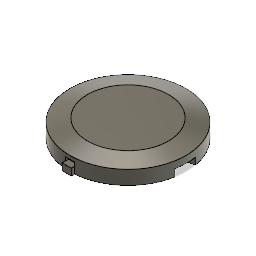
CaseBack (Autodesk Fusion 360 design; units mm, degrees)
Autodesk Fusion 360 part; units mm, degrees
sketch "Sketch1" plane through (0, 0, 0) normal (0, 1, 0) x (1, 0, 0)
  circle A0 centre (0, 0) radius 16.4
  dimension "d1" = 32.8
  measures "d1" diameter of A0
extrude "Extrude1" add sketch "Sketch1" along normal blind 5
chamfer "Chamfer1" distance 5 distance2 1 1 edges at (-15.2902, 5, 5.9305) measured on face at (3.2266, 5, -3.4774)
sketch "Sketch2" plane through (0, 0, 0) normal (1, 0, 0) x (0, 0, -1)
  line L0 (16.4, 0) -> (17.3, 0)
  line L1 (17.3, 0) -> (17.3, 2)
  line L2 (17.3, 2) -> (16.4, 2)
  line L3 (16.4, 2) -> (16.4, 0)
  line L4 (-16.4, 0) -> (-17.3, 0)
  line L5 (-17.3, 0) -> (-17.3, 2)
  line L6 (-17.3, 2) -> (-16.4, 2)
  line L7 (-16.4, 2) -> (-16.4, 0)
  dimension "d7" = 16.4
  dimension "d8" = 2
  dimension "d9" = 0.9
  dimension "d10" = 16.4
  dimension "d11" = 2
  dimension "d12" = 0.9
  measures "d7" distance of origin
  measures "d10" distance of origin
revolve "Revolve1" add sketch "Sketch2" angle 4.5 about axis through (0, 1.75, 0) along (0, 1, 0) second angle 4.5
sketch "Sketch3" plane through (0, 0, 0) normal (0, 1, 0) x (1, 0, 0)
  circle A0 centre (0, 0) radius 13.5
  dimension "d15" = 27
  measures "d15" diameter of A0
extrude "Extrude2" cut sketch "Sketch3" along normal blind 2.78
sketch "Sketch4" plane through (0, 0, 0) normal (0, 0, 1) x (1, 0, 0)
  line L0 (0, 0) -> (16.5, 0)
  line L1 (16.5, 0) -> (16.5, 2)
  line L2 (16.5, 2) -> (0, 2)
  line L3 (0, 2) -> (0, 0)
  dimension "d18" = 16.5
  dimension "d19" = 2
  measures "d18" distance of L0.start
  measures "d19" distance of L0.start
revolve "Revolve2" cut sketch "Sketch4" angle 10 about axis through (0, 1.75, 0) along (0, 1, 0) second angle 10
sketch "Sketch5" plane through (0, 0, 0) normal (1, 0, 0) x (0, 0, -1)
  line L0 (-16.5, 2) -> (-15.5, 2)
  line L1 (-15.5, 2) -> (-15.5, 3)
  line L2 (-15.5, 3) -> (-16.5, 3)
  line L3 (-16.5, 3) -> (-16.5, 2)
  line L4 (16.5, 0) -> (16.5, 2)
  line L5 (16.5, 2) -> (15.5, 2)
  line L6 (15.5, 2) -> (15.5, 3)
  line L7 (15.5, 3) -> (16.5, 3)
  line L8 (16.5, 3) -> (16.5, 2)
  dimension "d24" = 1
  dimension "d25" = 1
  dimension "d28" = 16.5
  dimension "d29" = 2
  dimension "d30" = 1
  dimension "d31" = 1
  measures "d28" distance of origin
revolve "Revolve4" cut sketch "Sketch5" angle 4.5 about axis through (0, 1.75, 0) along (0, 1, 0) second angle 4.5 contours L5 L6 L7 L8
revolve "Revolve3" cut sketch "Sketch5" angle 4.5 about axis through (0, 1.75, 0) along (0, 1, 0) second angle 4.5 contours L0 L1 L2 L3
